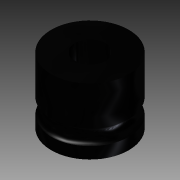
# Autodesk Inventor part: HOBBED PULLEY
Saved by Autodesk Inventor 2013 (Build 170138000, 138)
## iProperties
Created: 2013-12-22
Part Number: HOBBED PULLEY
Material: Generic
Document SubType Name: Modeling
Designer: employee
Density: 1 g/cm^3
Mass: 1.08885 g
Surface Area: 8.35685 cm^2
Volume: 1.08885 cm^3
Author: employee
Autodesk Inventor part; units mm, degrees
ref_plane "YZ Plane" through (0, 0, 0) normal (1, 0, 0) x (0, 1, 0)
ref_plane "XZ Plane" through (0, 0, 0) normal (0, 1, 0) x (-1, 0, 0)
ref_plane "XY Plane" through (0, 0, 0) normal (0, 0, 1) x (1, 0, 0)
sketch "Sketch1" plane through (0, 0, 0) normal (0, 1, 0) x (-1, 0, 0)
  line L0 (-2.5, 0) -> (-2.5, 10.795)
  line L1 (-2.5, 10.795) -> (-6.35, 10.795)
  line L2 (-6.35, 10.795) -> (-6.35, 4.445)
  arc A0 (-6.35, 1.905) -> (-6.35, 4.445) centre (-6.7204, 3.175) ccw
  line L3 (-6.35, 1.905) -> (-6.35, 0)
  line L4 (-6.35, 0) -> (-2.5, 0)
  line L5 (-6.7204, 3.175) -> (-5.3975, 3.175)
  line L6 (0, -2.159) -> (0, 12.954) projected
  point P0 (0, 0)
  dimension "d0" = 2.5
  dimension "d1" = 6.35
  dimension "d2" = 5.3975
  dimension "d3" = 10.795
  dimension "d4" = 7.62
  dimension "d5" = 2.54
  constraints: 12 end point, 3 point on circle, 2 perpendicular, 1 centre point, 1 collinear, 1 horizontal alignment, 1 parallel, 1 vertical, 1 vertical alignment
  measures "d0" distance from line of point (0, 0) L0
  measures "d1" distance from line of point (0, 0) L3
  measures "d2" horizontal distance of point (0, 0) L5.end
  measures "d3" distance between parallel lines of L4 L1
  measures "d4" distance from line of L5.start L1
  measures "d5" distance of L2.end L3.start
revolve "Revolution1" add sketch "Sketch1" angle 360 about axis through (0, 0, -10) along (0, 0, 1)
body "Solid1"
